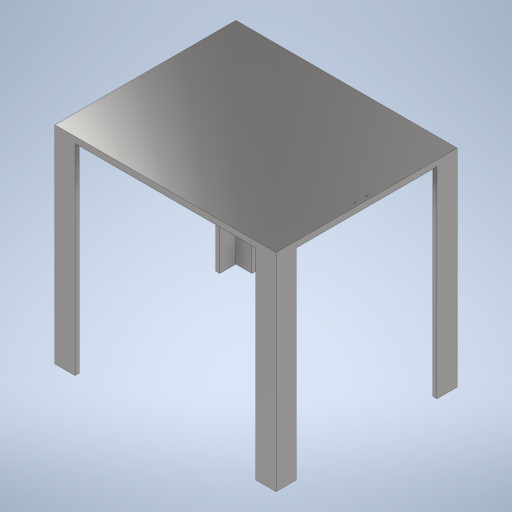
# Autodesk Inventor part: Work table
Saved by Autodesk Inventor 2024 (Build 280153020, 153B)
## iProperties
Created: 2023-08-29
Part Number: Work table
Material: Steel, Mild
Document SubType Name: Modeling
Designer: Victoria
Density: 7.85 g/cm^3
Appearance: Semi-Polished
Author: Victoria
Autodesk Inventor part; units mm, degrees
ref_plane "YZ Plane" through (0, 0, 0) normal (1, 0, 0) x (0, 1, 0)
ref_plane "XZ Plane" through (0, 0, 0) normal (0, 1, 0) x (-1, 0, 0)
ref_plane "XY Plane" through (0, 0, 0) normal (0, 0, 1) x (1, 0, 0)
sketch "Sketch1" plane through (0, 0, 0) normal (0, 1, 0) x (-1, 0, 0)
  line L0 (275, 225) -> (-275, 225)
  line L1 (-275, 225) -> (-275, -225)
  line L2 (-275, -225) -> (275, -225)
  line L3 (275, -225) -> (275, 225)
  line L4 (275, 225) -> (-275, -225) construction
  line L5 (-275, 225) -> (275, -225) construction
  point P0 (0, 0)
  dimension "d0" = 550
  dimension "d1" = 450
  constraints: 12 end point, 2 midpoint, 2 parallel, 1 horizontal, 1 perpendicular
  measures "d0" distance of L2.end L1.end
  measures "d1" distance of L1.end L0.end
extrude "Extrusion1" add sketch "Sketch1" against normal blind 15
sketch "Sketch2" plane through (0, -15, 0) normal (0, -1, 0) x (1, 0, 0)
  line L0 (275, -225) -> (275, 225) projected
  line L1 (275, 225) -> (225, 225)
  line L2 (225, 225) -> (225, 175)
  line L3 (225, 175) -> (275, 175)
  line L4 (275, 175) -> (275, 225)
  line L5 (-275, -225) -> (275, -225) projected
  line L6 (275, -225) -> (225, -225)
  line L7 (225, -225) -> (225, -175)
  line L8 (225, -175) -> (275, -175)
  line L9 (275, -175) -> (275, -225)
  line L10 (-275, 225) -> (-275, -225) projected
  line L11 (-275, -225) -> (-225, -225)
  line L12 (-225, -225) -> (-225, -175)
  line L13 (-225, -175) -> (-275, -175)
  line L14 (-275, -175) -> (-275, -225)
  line L15 (-275, 225) -> (-225, 225)
  line L16 (-225, 225) -> (-225, 175)
  line L17 (-225, 175) -> (-275, 175)
  line L18 (-275, 175) -> (-275, 225)
  point P0 (0, 0)
  dimension "d4" = 50
  dimension "d5" = 50
  dimension "d6" = 50
  dimension "d7" = 50
  constraints: 32 end point, 8 parallel, 4 horizontal, 4 perpendicular, 4 point on line
  measures "d4" distance of L3.end L2.end
  measures "d5" distance of L2.end L1.end
  measures "d6" distance of L6.end L7.end
  measures "d7" distance of L13.end L12.end
extrude "Extrusion2" add sketch "Sketch2" along normal blind 500
sketch "Sketch3" plane through (0, -515, 0) normal (0, -1, 0) x (1, 0, 0)
  line L0 (225, 175) -> (275, 175) projected
  line L1 (225, 175) -> (265, 175)
  line L2 (265, 175) -> (265, 215)
  line L3 (265, 215) -> (225, 215)
  line L4 (225, 215) -> (225, 175)
  point P0 (0, 0)
  dimension "d10" = 40
  dimension "d11" = 40
  constraints: 8 end point, 2 parallel, 1 horizontal, 1 perpendicular
  measures "d10" distance of L3.end L2.end
  measures "d11" distance of L2.end L1.end
extrude "Extrusion3" cut sketch "Sketch3" against normal blind 500
mirror "Mirror1" about plane through (0, 0, 0) normal (1, 0, 0) of "Extrusion3"
mirror "Mirror2" about plane through (0, 0, 0) normal (0, 0, 1) of "Extrusion3"
sketch "Sketch4" plane through (0, -515, 0) normal (0, -1, 0) x (1, 0, 0)
  line L0 (-275, -175) -> (-225, -175) projected
  line L1 (-225, -175) -> (-265, -175)
  line L2 (-265, -175) -> (-265, -215)
  line L3 (-265, -215) -> (-225, -215)
  line L4 (-225, -215) -> (-225, -175)
  point P0 (0, 0)
  dimension "d14" = 40
  dimension "d15" = 40
  constraints: 8 end point, 2 parallel, 1 horizontal, 1 perpendicular
  measures "d14" distance of L3.end L2.end
  measures "d15" distance of L2.end L1.end
extrude "Extrusion4" cut sketch "Sketch4" against normal blind 500
sketch "Sketch5" plane through (0, 0, 0) normal (0, 1, 0) x (1, 0, 0)
  line L0 (275, -225) -> (275, 225) projected
  line L1 (275, 0) -> (265, 0)
  line L2 (265, 0) -> (265, -19.5)
  line L3 (265, -19.5) -> (265, 9.5)
  circle A0 centre (265, 9.5) radius 2.5
  circle A1 centre (265, -19.5) radius 2.5
  point P0 (0, 0)
  dimension "d18" = 10
  dimension "d19" = 19.5
  dimension "d20" = 29
  dimension "d21" = 5
  dimension "d22" = 5
  constraints: 6 end point, 2 centre point, 2 coincident, 1 horizontal, 1 midpoint, 1 perpendicular, 1 point on line
  measures "d18" distance of L1.start L1.end
  measures "d19" distance of L1.end L2.end
  measures "d20" distance of L2.end L3.end
  measures "d21" diameter of A0
  measures "d22" diameter of A1
extrude "Extrusion5" cut sketch "Sketch5" against normal through all
thread "Thread1" size "M5x0.8" class "6H" standard "ISO Metric profile" full length
thread "Thread2" size "M5x0.8" class "6H" standard "ISO Metric profile" full length
ref_plane "Work Plane1" through (0, 0, 0) normal (1, 0, 0) x (0, 1, 0)
ref_plane "Work Plane2" through (0, 0, 0) normal (0, 0, 1) x (1, 0, 0)
body "Solid1"
